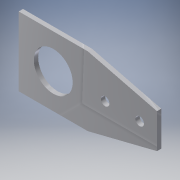
# Autodesk Inventor part: Wheel Gusset
Saved by Autodesk Inventor 2016 (Build 200138000, 138)
## iProperties
Created: 2016-01-17
Part Number: Wheel Gusset
Material: Aluminum 6061
Document SubType Name: Modeling
Designer: gus
Density: 2.7 g/cm^3
Appearance: Aluminum - Flat
Mass: 32.6739 g
Surface Area: 89.3168 cm^2
Volume: 12.1014 cm^3
Author: gus
Autodesk Inventor part; units mm, degrees
ref_plane "YZ Plane" through (0, 0, 0) normal (1, 0, 0) x (0, 1, 0)
ref_plane "XZ Plane" through (0, 0, 0) normal (0, 1, 0) x (-1, 0, 0)
ref_plane "XY Plane" through (0, 0, 0) normal (0, 0, 1) x (1, 0, 0)
sketch "Sketch1" plane through (0, 0, 0) normal (0, 0, 1) x (1, 0, 0)
  line L0 (0, 0) -> (-50.8, 12.7)
  line L1 (-50.8, 12.7) -> (-101.6, 12.7)
  line L2 (-101.6, 12.7) -> (-101.6, -38.1)
  line L3 (-101.6, -38.1) -> (-50.8, -38.1)
  line L4 (-50.8, -38.1) -> (0, -25.4)
  line L5 (0, -25.4) -> (0, 0)
  circle A0 centre (-76.2, -12.7) radius 14.2875
  circle A1 centre (-12.7, -12.7) radius 3.175
  circle A2 centre (-38.1, -12.7) radius 3.175
  line L6 (-101.6, -12.7) -> (0, -12.7) construction
  dimension "d1" = 50.8
  dimension "d2" = 50.8
  dimension "d3" = 50.8
  dimension "d4" = 25.4
  dimension "d5" = 28.575
  dimension "d6" = 25.4
  dimension "d7" = 25.4
  dimension "d8" = 6.35
  dimension "d9" = 6.35
  dimension "d10" = 12.7
  dimension "d11" = 25.4
  constraints: 14 end point, 3 centre point, 2 equal length, 2 midpoint, 2 parallel, 2 point on line, 1 coincident, 1 horizontal, 1 perpendicular
  measures "d1" distance of L0.end L1.end
  measures "d2" distance of L1.end L2.end
  measures "d3" distance from line of L3.end L5
  measures "d4" distance of L4.end L0.start
  measures "d5" diameter of A0
  measures "d6" distance from line of L3 A0.centre
  measures "d7" distance from line of L2 A0.centre
  measures "d8" diameter of A1
  measures "d9" diameter of A2
  measures "d10" distance from line of L5 A1.centre
  measures "d11" distance of A2.centre A1.centre
extrude "Extrusion1" add sketch "Sketch1" along normal blind 3.175
body "Solid1"
